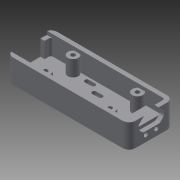
# Autodesk Inventor part: dualBaccable-ucan_fysect
Saved by Autodesk Inventor 2014 SP2 (Build 180246200, 246)
## iProperties
Created: 2025-01-14
Part Number: dualBaccable-ucan_fysect
Material: Generic
Document SubType Name: Sheet Metal
Designer: GauchoHP
Density: 1 g/cm^3
Sheet Metal Rule: Default_mm
Appearance: Default
Author: GauchoHP
Autodesk Inventor part; units mm, degrees
ref_plane "YZ Plane" through (0, 0, 0) normal (1, 0, 0) x (0, 1, 0)
ref_plane "XZ Plane" through (0, 0, 0) normal (0, 1, 0) x (-1, 0, 0)
ref_plane "XY Plane" through (0, 0, 0) normal (0, 0, 1) x (1, 0, 0)
sketch "Sketch1" plane through (0, 0, 0) normal (0, 0, 1) x (1, 0, 0)
  line L0 (-27.1053, 8.3421) -> (24.8947, 8.3421)
  line L1 (27.8947, 5.3421) -> (27.8947, -9.6579)
  line L2 (24.8947, -12.6579) -> (-27.1053, -12.6579)
  line L3 (-30.1053, -9.6579) -> (-30.1053, 5.3421)
  arc A0 (-27.1053, 8.3421) -> (-30.1053, 5.3421) centre (-27.1053, 5.3421) ccw
  arc A1 (27.8947, 5.3421) -> (24.8947, 8.3421) centre (24.8947, 5.3421) ccw
  arc A2 (24.8947, -12.6579) -> (27.8947, -9.6579) centre (24.8947, -9.6579) ccw
  arc A3 (-30.1053, -9.6579) -> (-27.1053, -12.6579) centre (-27.1053, -9.6579) ccw
  point P0 (0, 0)
  point P1 (-30.1053, 8.3421)
  point P2 (27.8947, 8.3421)
  point P3 (-30.1053, -12.6579)
  dimension "d0" = 21
  dimension "d1" = 58
  dimension "d2" = 3
  constraints: 8 end point, 8 point on circle, 8 tangent, 6 point on line, 4 centre point, 3 equal radius, 2 parallel, 1 horizontal, 1 perpendicular
  measures "d0" distance of point (-30.105, -12.658) point (-30.105, 8.342)
  measures "d1" distance of point (-30.105, 8.342) point (27.895, 8.342)
  measures "d2" radius of A0
extrude "Extrusion1" add sketch "Sketch1" along normal blind 2
sketch "Sketch2" plane through (0, 0, 2) normal (0, 0, 1) x (1, 0, 0)
  line L0 (24.8947, 8.3421) -> (-27.1053, 8.3421) projected
  arc A0 (-27.1053, 8.3421) -> (-30.1053, 5.3421) centre (-27.1053, 5.3421) ccw projected
  line L1 (-30.1053, 5.3421) -> (-30.1053, -9.6579) projected
  arc A1 (-30.1053, -9.6579) -> (-27.1053, -12.6579) centre (-27.1053, -9.6579) ccw projected
  line L2 (-27.1053, -12.6579) -> (24.8947, -12.6579) projected
  arc A2 (24.8947, -12.6579) -> (27.8947, -9.6579) centre (24.8947, -9.6579) ccw projected
  line L3 (27.8947, -9.6579) -> (27.8947, 5.3421) projected
  arc A3 (27.8947, 5.3421) -> (24.8947, 8.3421) centre (24.8947, 5.3421) ccw projected
  line L4 (-27.1053, 6.3421) -> (24.8947, 6.3421)
  arc A4 (25.8947, 5.3421) -> (24.8947, 6.3421) centre (24.8947, 5.3421) ccw
  line L5 (25.8947, 5.3421) -> (25.8947, -9.6579)
  arc A5 (24.8947, -10.6579) -> (25.8947, -9.6579) centre (24.8947, -9.6579) ccw
  line L6 (24.8947, -10.6579) -> (-27.1053, -10.6579)
  arc A6 (-28.1053, -9.6579) -> (-27.1053, -10.6579) centre (-27.1053, -9.6579) ccw
  line L7 (-28.1053, -9.6579) -> (-28.1053, 5.3421)
  arc A7 (-27.1053, 6.3421) -> (-28.1053, 5.3421) centre (-27.1053, 5.3421) ccw
  point P0 (0, 0)
  dimension "d5" = 2
  constraints: 8 end point, 8 point on circle, 4 centre point, 7 other
  measures "d5" distance between parallel lines of L4 L0
extrude "Extrusion2" add sketch "Sketch2" along normal blind 9.2
sketch "Sketch4" plane through (-28.1053, -9.6579, 2) normal (1, 0, 0) x (0, 0, -1)
  line L0 (0, 15) -> (0, 0) projected
  line L1 (0, 15) -> (-9.2, 15) projected
  line L2 (0, 0) -> (-9.2, 0) projected
  line L3 (0, 13) -> (-9.5, 13)
  line L4 (-9.5, 13) -> (-9.5, 0)
  line L5 (-9.5, 0) -> (0, 0)
  line L6 (0, 0) -> (0, 13)
  line L7 (-9.5, -1) -> (-7.5, -1)
  line L8 (-7.5, -1) -> (-7.5, 16)
  line L9 (-7.5, 16) -> (-9.5, 16)
  line L10 (-9.5, 16) -> (-9.5, -1)
  point P0 (2, 9.6579)
  dimension "d22" = 9.5
  dimension "d23" = 13
  dimension "d26" = 0
  dimension "d27" = 2
  dimension "d28" = 1
  dimension "d29" = 17
  dimension "d30" = 1
  dimension "d31" = 1
  dimension "d32" = 3
  dimension "d53" = 0
  constraints: 16 end point, 4 parallel, 2 horizontal, 2 perpendicular, 1 point on line
  measures "d22" distance of L5.end L4.end
  measures "d23" distance of L4.end L3.end
  measures "d26" distance between parallel lines of L5 L2
  measures "d27" distance of L8.end L9.end
  measures "d28" distance between parallel lines of L5 L7
  measures "d29" distance of L9.end L7.start
  measures "d30" distance between parallel lines of L9 L1
  measures "d31" distance between parallel lines of L2 L7
  measures "d32" distance between parallel lines of L9 L3
  measures "d53" distance between parallel lines of L4 L10
extrude "Extrusion4" cut sketch "Sketch4" along normal mid plane 10 contours L0 L2 L8 L3 | L8 L3 L10 L9 | L8 L2 L5 L4 L3 | L8 L7 L10 L5 L2
sketch "Sketch5" plane through (0, 0, 2) normal (0, 0, 1) x (1, 0, 0)
  line L0 (-27.1053, -10.6579) -> (24.8947, -10.6579) projected
  line L1 (25.8947, -9.6579) -> (25.8947, 5.3421) projected
  line L2 (24.8947, 6.3421) -> (-27.1053, 6.3421) projected
  line L3 (18.8947, 4.3421) -> (25.8947, 4.3421)
  line L4 (25.8947, 4.3421) -> (25.8947, -8.6579)
  line L5 (25.8947, -8.6579) -> (18.8947, -8.6579)
  line L6 (18.8947, -8.6579) -> (18.8947, 4.3421)
  point P0 (0, 0)
  dimension "d35" = 0
  dimension "d36" = 13
  dimension "d37" = 2
  dimension "d38" = 2
  dimension "d39" = 7
  constraints: 8 end point, 2 parallel, 1 horizontal, 1 perpendicular
  measures "d35" distance between parallel lines of L1 L4
  measures "d36" distance of L5.end L3.start
  measures "d37" distance between parallel lines of L2 L3
  measures "d38" distance between parallel lines of L0 L5
  measures "d39" distance of L3.start L3.end
extrude "Extrusion5" add sketch "Sketch5" along normal blind 4
sketch "Sketch6" plane through (0, 0, 2) normal (0, 0, 1) x (1, 0, 0)
  line L0 (25.8947, 4.3421) -> (25.8947, 5.3421) projected
  line L1 (24.8947, 6.3421) -> (-27.1053, 6.3421) projected
  line L2 (-27.1053, -10.6579) -> (24.8947, -10.6579) projected
  line L3 (25.8947, -9.6579) -> (25.8947, -8.6579) projected
  circle A0 centre (14.8947, 4.3421) radius 2.5
  circle A1 centre (14.8947, -8.6579) radius 2.5
  circle A2 centre (14.8947, 4.3421) radius 1
  circle A3 centre (14.8947, -8.6579) radius 1
  circle A4 centre (-15.6053, 4.3421) radius 2.5
  circle A5 centre (-15.6053, -8.6579) radius 2.5
  circle A6 centre (-15.6053, 4.3421) radius 1
  circle A7 centre (-15.6053, -8.6579) radius 1
  point P0 (0, 0)
  dimension "d42" = 5
  dimension "d43" = 5
  dimension "d44" = 11
  dimension "d45" = 11
  dimension "d46" = 2
  dimension "d47" = 2
  dimension "d48" = 13
  dimension "d49" = 2
  dimension "d50" = 2
  dimension "d61" = 5
  dimension "d62" = 5
  dimension "d63" = 2
  dimension "d64" = 2
  dimension "d65" = 13
  dimension "d66" = 2
  dimension "d67" = 30.5
  constraints: 8 centre point, 4 coincident
  measures "d42" diameter of A0
  measures "d43" diameter of A1
  measures "d44" distance from line of A1.centre L3
  measures "d45" distance from line of L0 A0.centre
  measures "d46" diameter of A2
  measures "d47" diameter of A3
  measures "d48" distance of A0.centre A1.centre
  measures "d49" distance from line of L1 A2.centre
  measures "d50" distance from line of L2 A1.centre
  measures "d61" diameter of A4
  measures "d62" diameter of A5
  measures "d63" diameter of A6
  measures "d64" diameter of A7
  measures "d65" distance of A4.centre A5.centre
  measures "d66" distance from line of L1 A6.centre
  measures "d67" distance of A0.centre A4.centre
extrude "Extrusion6" add sketch "Sketch6" along normal blind 7.5
sketch "Sketch7" plane through (14.8947, -8.6579, 2) normal (0, 0, 1) x (1, 0, 0)
  circle A0 centre (0, 0) radius 1 projected
  point P0 (-14.8947, 8.6579)
extrude "Extrusion7" cut sketch "Sketch7" against normal blind 7
sketch "Sketch8" plane through (14.8947, 4.3421, 2) normal (0, 0, 1) x (1, 0, 0)
  circle A0 centre (0, 0) radius 1 projected
  point P0 (-14.8947, -4.3421)
extrude "Extrusion8" cut sketch "Sketch8" against normal blind 7
sketch "Sketch9" plane through (-15.6053, 4.3421, 2) normal (0, 0, 1) x (1, 0, 0)
  circle A0 centre (0, 0) radius 1 projected
  point P0 (15.6053, -4.3421)
extrude "Extrusion9" cut sketch "Sketch9" against normal blind 7
sketch "Sketch10" plane through (-15.6053, -8.6579, 2) normal (0, 0, 1) x (1, 0, 0)
  circle A0 centre (0, 0) radius 1 projected
  point P0 (15.6053, 8.6579)
extrude "Extrusion10" cut sketch "Sketch10" against normal blind 7
chamfer "Chamfer1" distance 2 angle 45 4 edges at (13.8947, -8.6579, 0) (13.8947, 4.3421, 0) (-16.6053, 4.3421, 0) (-16.6053, -8.6579, 0)
sketch "Sketch11" plane through (25.8947, -9.6579, 11.2) normal (-1, 0, 0) x (0, 0, 1)
  line L0 (-9.2, 0) -> (0, 0) projected
  line L1 (-9.2, 15) -> (0, 15) projected
  line L2 (0, 11.0554) -> (-2.4966, 13.552)
  line L3 (-4.1682, 13.552) -> (-2.4966, 13.552)
  arc A0 (-4.1682, 13.552) -> (-5.2824, 12.9662) centre (-3.8419, 11.5788) ccw
  arc A1 (-6.1108, 12.1378) -> (-6.6966, 10.7236) centre (-4.6966, 10.7236) ccw
  line L4 (-5.2824, 12.9662) -> (-6.1108, 12.1378)
  arc A2 (-6.6966, 4.3804) -> (-6.1108, 2.9662) centre (-4.6966, 4.3804) ccw
  line L5 (-6.1108, 2.9662) -> (-5.2824, 2.1378)
  line L6 (-2.4966, 1.552) -> (-4.1682, 1.552)
  line L7 (-2.4966, 1.552) -> (0, 4.0486)
  arc A3 (-5.2824, 2.1378) -> (-4.1682, 1.552) centre (-3.8419, 3.5252) ccw
  line L8 (-6.6966, 10.7236) -> (-6.6966, 4.3804)
  line L9 (-5.2, 1) -> (-9.2, 1) projected
  line L10 (-5.2, 14) -> (-5.2, 1) projected
  line L11 (-5.2, 1) -> (-6.7, 1)
  line L12 (0, 15) -> (0, 0) projected
  line L13 (0, 11.0554) -> (0, 4.0486)
  point P0 (-11.2, 9.6579)
  point P1 (-0.4966, 11.552)
  point P2 (-0.4966, 3.552)
  dimension "d72" = 1.448
  dimension "d73" = 1.552
  dimension "d77" = 1.5
  dimension "d78" = 1.4966
  constraints: 18 end point, 8 point on circle, 5 point on line, 4 centre point, 2 tangent, 1 collinear
  measures "d72" distance between parallel lines of L1 L3
  measures "d73" distance between parallel lines of L0 L6
  measures "d77" distance of L9.start L11.end
  measures "d78" distance between parallel lines of L10 L8
extrude "Extrusion11" cut sketch "Sketch11" against normal blind 7
sketch "Sketch12" plane through (27.8947, -9.6579, 0) normal (1, 0, 0) x (0, 0, -1)
  line L0 (0, 15) -> (0, 0) projected
  line L1 (0, 15) -> (-11.2, 15) projected
  line L2 (0, 0) -> (-11.2, 0) projected
  circle A0 centre (-3, 10) radius 1
  circle A1 centre (-3, 5) radius 1
  point P0 (0, 9.6579)
  dimension "d79" = 2
  dimension "d80" = 2
  dimension "d81" = 3
  dimension "d82" = 3
  dimension "d83" = 5
  dimension "d84" = 5
  constraints: 2 centre point
  measures "d79" diameter of A0
  measures "d80" diameter of A1
  measures "d81" distance from line of L0 A1.centre
  measures "d82" distance from line of L0 A0.centre
  measures "d83" distance from line of L2 A1.centre
  measures "d84" distance from line of L1 A0.centre
extrude "Extrusion12" cut sketch "Sketch12" against normal blind 10
sketch "Sketch13" plane through (0, 0, 2) normal (0, 0, 1) x (1, 0, 0)
  line L0 (25.8947, 4.3421) -> (25.8947, 5.3421) projected
  line L1 (13.3947, 6.3421) -> (-14.1053, 6.3421) projected
  line L2 (-2.6053, 2.3421) -> (0.3947, 2.3421)
  line L3 (1.3947, 1.3421) -> (1.3947, 1.3421)
  line L4 (0.3947, 0.3421) -> (-2.6053, 0.3421)
  line L5 (-3.6053, 1.3421) -> (-3.6053, 1.3421)
  arc A0 (-2.6053, 2.3421) -> (-3.6053, 1.3421) centre (-2.6053, 1.3421) ccw
  arc A1 (1.3947, 1.3421) -> (0.3947, 2.3421) centre (0.3947, 1.3421) ccw
  arc A2 (0.3947, 0.3421) -> (1.3947, 1.3421) centre (0.3947, 1.3421) ccw
  arc A3 (-3.6053, 1.3421) -> (-2.6053, 0.3421) centre (-2.6053, 1.3421) ccw
  line L6 (-9.1053, 5.3421) -> (-6.1053, 5.3421)
  line L7 (-5.1053, 4.3421) -> (-5.1053, 4.3421)
  line L8 (-6.1053, 3.3421) -> (-9.1053, 3.3421)
  line L9 (-10.1053, 4.3421) -> (-10.1053, 4.3421)
  arc A4 (-9.1053, 5.3421) -> (-10.1053, 4.3421) centre (-9.1053, 4.3421) ccw
  arc A5 (-5.1053, 4.3421) -> (-6.1053, 5.3421) centre (-6.1053, 4.3421) ccw
  arc A6 (-6.1053, 3.3421) -> (-5.1053, 4.3421) centre (-6.1053, 4.3421) ccw
  arc A7 (-10.1053, 4.3421) -> (-9.1053, 3.3421) centre (-9.1053, 4.3421) ccw
  point P0 (0, 0)
  point P1 (-3.6053, 2.3421)
  point P2 (1.3947, 2.3421)
  point P3 (-3.6053, 0.3421)
  point P4 (1, 1)
  point P5 (-10.1053, 5.3421)
  point P6 (-5.1053, 5.3421)
  point P7 (-10.1053, 3.3421)
  dimension "d87" = 24.5
  dimension "d88" = 5
  dimension "d89" = 4
  dimension "d90" = 2
  dimension "d91" = 1
  dimension "d97" = 5
  dimension "d98" = 2
  dimension "d99" = 1
  dimension "d100" = 1
  dimension "d101" = 32
  constraints: 16 end point, 16 point on circle, 16 tangent, 12 point on line, 8 centre point, 6 equal radius, 4 parallel, 2 horizontal, 2 perpendicular
  measures "d87" distance between parallel lines of L3 L0
  measures "d88" distance of point (-3.605, 2.342) point (1.395, 2.342)
  measures "d89" distance between parallel lines of L1 L2
  measures "d90" distance of point (-3.605, 0.342) point (-3.605, 2.342)
  measures "d91" radius of A0
  measures "d97" distance of point (-10.105, 5.342) point (-5.105, 5.342)
  measures "d98" distance of point (-10.105, 3.342) point (-10.105, 5.342)
  measures "d99" radius of A4
  measures "d100" distance between parallel lines of L1 L6
  measures "d101" distance from line of L0 A5.centre
extrude "Extrusion13" cut sketch "Sketch13" against normal blind 10
chamfer "Chamfer2" distance 0.5 angle 45 8 edges at (-1.1053, 0.3421, 0) (1.3947, 1.3421, 0) (-1.1053, 2.3421, 0) (-3.6053, 1.3421, 0) (-7.6053, 3.3421, 0) (-5.1053, 4.3421, 0) (-7.6053, 5.3421, 0) (-10.1053, 4.3421, 0)
equation "\"BendRadius\" = Thickness"
equation "\"BendReliefWidth\" = Thickness"
equation "\"BendReliefDepth\" = 0.5 * Thickness"
equation "\"CornerReliefSize\" = 4 * Thickness"
equation "\"MinimumRemnant\" = 2 * Thickness"
equation "\"TransitionRadius\" = BendRadius"
equation "\"JacobiRadiusSize\" = BendRadius"
equation "\"GapSize\" = Thickness"
equation "\"Thickness\" = 0.5"
body "Solid1"
